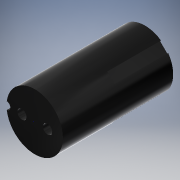
# Autodesk Inventor part: center_2p_female_body
Saved by Autodesk Inventor 2018 (Build 220112000, 112)
## iProperties
Created: 2019-04-17
Part Number: center_2p_female_body
Material: Generic
Document SubType Name: Modeling
Designer: ZEUSLAP
Density: 1 g/cm^3
Appearance: Default
Author: ZEUSLAP
Autodesk Inventor part; units mm, degrees
ref_plane "YZ Plane" through (0, 0, 0) normal (1, 0, 0) x (0, 1, 0)
ref_plane "XZ Plane" through (0, 0, 0) normal (0, 1, 0) x (-1, 0, 0)
ref_plane "XY Plane" through (0, 0, 0) normal (0, 0, 1) x (1, 0, 0)
sketch "Sketch1" plane through (0, 0, 0) normal (0, 1, 0) x (-1, 0, 0)
  arc A0 (5.4489, 0.7483) -> (5.4489, -0.7483) centre (0, 0) ccw
  arc A1 (5.4489, 0.7483) -> (5.4489, -0.7483) centre (5.5, 0) ccw
  dimension "d0" = 11
  dimension "d1" = 1.5
  constraints: 5 point on circle, 2 centre point, 1 coincident
  measures "d0" diameter of A0
  measures "d1" diameter of A1
extrude "Extrusion1" add sketch "Sketch1" along normal blind 11
sketch "Sketch2" plane through (0, 11, 0) normal (0, 1, 0) x (1, 0, 0)
  line L0 (-4.9, -2.498) -> (-3.7228, -4.8072) construction
  line L1 (-4.9, -2.498) -> (-4.7307, -2.3916)
  line L2 (-4.9089, 2.4924) -> (-3.4167, 5.4194) construction
  line L3 (-4.9089, 2.4924) -> (-4.7307, 2.4016)
  line L4 (-4.7307, 2.4016) -> (-4.7307, 1.1516) construction
  line L5 (-4.7307, 2.4016) -> (-4.9089, 1.1516)
  line L6 (-4.9089, 1.1516) -> (-4.7307, -0.0056)
  line L7 (-4.7307, -2.3916) -> (-4.7307, -1.1416) construction
  line L8 (-4.7307, -2.3916) -> (-4.9089, -1.1627)
  line L9 (-4.9089, -1.1627) -> (-4.7307, -0.0056)
  arc A0 (-4.9, -2.498) -> (3.1172, -4.5314) centre (0, 0) ccw
  arc A1 (4.5314, -3.1172) -> (4.5314, 3.1172) centre (0, 0) ccw
  arc A2 (3.1202, 4.5358) -> (-4.9089, 2.4924) centre (0, 0) ccw
  line L10 (3.1172, -4.5314) -> (2.9345, -4.3487)
  line L11 (4.3487, -2.9345) -> (4.5314, -3.1172)
  line L12 (4.5314, 3.1172) -> (4.3524, 2.9382)
  line L13 (2.9375, 4.3531) -> (3.1202, 4.5358)
  line L14 (2.9345, -4.3487) -> (4.3487, -2.9345)
  line L15 (4.3524, 2.9382) -> (2.9375, 4.3531)
  dimension "d7" = 0.2
  dimension "d8" = 0.2
  dimension "d9" = 1.25
  dimension "d11" = 1.25
  constraints: 33 end point, 6 point on circle, 3 centre point, 2 perpendicular, 1 coincident, 1 vertical
  measures "d7" distance of L1.end L0.start
  measures "d8" distance of L2.start L3.end
  measures "d9" distance of L3.end L4.end
  measures "d11" distance of L1.end L7.end
extrude "Extrusion2" add sketch "Sketch2" along normal blind 10.5
sketch "Sketch3" plane through (0, 21.5, 0) normal (0, 1, 0) x (1, 0, 0)
  circle A0 centre (-2.5, 0) radius 0.9
  circle A1 centre (2.5, 0) radius 0.9
  point P0 (0, 0)
  dimension "d20" = 1.8
  dimension "d21" = 1.8
  dimension "d22" = 5
  dimension "d23" = 2.5
  constraints: 2 centre point
  measures "d20" diameter of A0
  measures "d21" diameter of A1
  measures "d22" distance of A1.centre A0.centre
  measures "d23" distance of point (0, 0) A0.centre
extrude "Extrusion3" cut sketch "Sketch3" against normal up to surface (21.5 mm away)
sketch "Sketch4" plane through (0, 0, 0) normal (0, -1, 0) x (1, 0, 0)
  line L0 (0, 0) -> (-0.2465, 0) construction
  constraints: 2 end point, 1 horizontal
body "Solid1"
